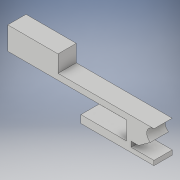
# Autodesk Inventor part: Halterung_MobileWhiteboard_V3_Ultrasonic scanner
Saved by Autodesk Inventor 2017 (Build 210142000, 142)
## iProperties
Part Number: Halterung_MobileWhiteboard_V3_Ultrasonic scanner
Material: Generisch
Document SubType Name: Modeling
Designer: Christoph Gürtner
Density: 1 g/cm^3
Appearance: Vorgabe
Author: Christoph Gürtner
Autodesk Inventor part; units mm, degrees
ref_plane "YZ Plane" through (0, 0, 0) normal (1, 0, 0) x (0, 1, 0)
ref_plane "XZ Plane" through (0, 0, 0) normal (0, 1, 0) x (-1, 0, 0)
ref_plane "XY Plane" through (0, 0, 0) normal (0, 0, 1) x (1, 0, 0)
sketch "Skizze1" plane through (0, 0, 0) normal (0, 1, 0) x (-1, 0, 0)
  arc A0 (4, -6.9282) -> (0, 8) centre (0, 0) ccw
  line L0 (0, -22) -> (0, -27)
  line L1 (0, -27) -> (30, -27)
  line L2 (80, 8) -> (0, 8)
  line L3 (0, -22) -> (25, -22)
  line L4 (25, -22) -> (0, -22)
  line L5 (25, -22) -> (25, -16.2)
  line L6 (25, -16) -> (25, -22)
  line L7 (25, -16.2) -> (16.7663, -16.2)
  line L8 (16.7663, -16.2) -> (4, -6.9282)
  line L9 (30, -27) -> (80, -27)
  line L10 (80, -27) -> (80, -18.6)
  line L11 (80, -18.6) -> (30, -18.6)
  line L12 (80, 1.45) -> (30, 1.45)
  line L13 (30, -18.6) -> (30, 1.45)
  line L14 (80, 1.45) -> (160, 1.45)
  line L15 (80, 1.45) -> (160, 1.45) construction
  line L16 (160, 1.45) -> (160, 26.45)
  line L17 (160, 26.45) -> (105, 26.45)
  line L18 (80, 8) -> (105, 8)
  line L19 (105, 8) -> (105, 26.45)
  circle A1 centre (119.5, 13.95) radius 8.025
  circle A2 centre (145.5, 13.95) radius 8.025
  dimension "d0" = 5
  dimension "d9" = 50
  dimension "d10" = 8.4
  dimension "d12" = 20.05
  dimension "d17" = 0
  dimension "d18" = 25
  dimension "d19" = 55
  dimension "d20" = 160
  dimension "d21" = 8
  dimension "d22" = 30
  dimension "d23" = 16.05
  dimension "d24" = 16.05
  dimension "d25" = 12.5
  dimension "d26" = 12.5
  dimension "d28" = 26
  dimension "d29" = 14.5
  constraints: 40 end point, 8 perpendicular, 7 horizontal, 3 centre point, 3 vertical, 2 point on circle, 1 coincident, 1 collinear, 1 point on line, 2 other
  measures "d0" distance of L0.start L0.end
  measures "d9" distance of L1.end L9.end
  measures "d10" distance of L9.end L10.end
  measures "d12" distance between parallel lines of L12 L11
  measures "d17" distance between parallel lines of L14 L15
  measures "d18" distance of L14.end L16.end
  measures "d19" distance of L16.end L17.end
  measures "d20" distance from line of L16 point (0, 0)
  measures "d21" distance from line of L2 point (0, 0)
  measures "d22" distance from line of L13 point (0, 0)
  measures "d23" diameter of A1
  measures "d24" diameter of A2
  measures "d25" distance from line of L15 A1.centre
  measures "d26" distance from line of L14 A2.centre
  measures "d28" distance of A2.centre A1.centre
  measures "d29" distance from line of A2.centre L16
extrude "Extrusion1" add sketch "Skizze1" along normal blind 20 contours A0 L2 L18 L19 L17 L16 L14 L12 L13 L11 L10 L9 L1 L0 L3 L5 L7 L8 | A1 | A2
